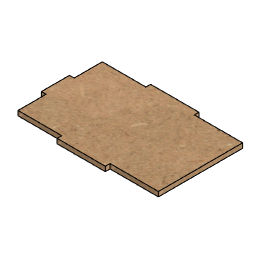
side step v13 (Autodesk Fusion 360 design; units mm, degrees)
Autodesk Fusion 360 part; units mm, degrees
sketch "Sketch1" plane through (0, 0, 0) normal (0, 0, 1) x (1, 0, 0)
  line L0 (-46.5, 30) -> (46.5, 30)
  line L1 (46.5, 30) -> (46.5, -30)
  line L2 (46.5, -30) -> (-46.5, -30)
  line L3 (-46.5, -30) -> (-46.5, 30)
  line L4 (-46.5, 30) -> (46.5, -30) construction
  line L5 (46.5, 30) -> (-46.5, -30) construction
  line L6 (-46.5, 30) -> (-15.5, 30)
  line L7 (-15.5, 30) -> (-15.5, 27)
  line L8 (-15.5, 27) -> (-46.5, 27)
  line L9 (-46.5, 27) -> (-46.5, 30)
  line L10 (-46.5, -30) -> (-15.5, -30)
  line L11 (-15.5, -30) -> (-15.5, -27)
  line L12 (-15.5, -27) -> (-46.5, -27)
  line L13 (-46.5, -27) -> (-46.5, -30)
  line L14 (46.5, 30) -> (15.5, 30)
  line L15 (15.5, 30) -> (15.5, 27)
  line L16 (15.5, 27) -> (46.5, 27)
  line L17 (46.5, 27) -> (46.5, 30)
  line L18 (46.5, -30) -> (15.5, -30)
  line L19 (15.5, -30) -> (15.5, -27)
  line L20 (15.5, -27) -> (46.5, -27)
  line L21 (46.5, -27) -> (46.5, -30)
  line L22 (46.5, 30) -> (43.5, 30)
  line L23 (43.5, 30) -> (43.5, 27)
  line L24 (43.5, 27) -> (46.5, 27)
  line L25 (46.5, 27) -> (46.5, 30)
  line L26 (46.5, -30) -> (43.5, -30)
  line L27 (43.5, -30) -> (43.5, -27)
  line L28 (43.5, -27) -> (46.5, -27)
  line L29 (46.5, -27) -> (46.5, -30)
  line L30 (-46.5, 27) -> (-43.5, 27)
  line L31 (-43.5, 27) -> (-43.5, 9)
  line L32 (-43.5, 9) -> (-46.5, 9)
  line L33 (-46.5, 9) -> (-46.5, 27)
  line L34 (-46.5, -27) -> (-43.5, -27)
  line L35 (-43.5, -27) -> (-43.5, -9)
  line L36 (-43.5, -9) -> (-46.5, -9)
  line L37 (-46.5, -9) -> (-46.5, -27)
  dimension "d1" = 93
  dimension "d2" = 60
  dimension "d3" = 31
  dimension "d4" = 3
  dimension "d5" = 31
  dimension "d6" = 3
  dimension "d7" = 31
  dimension "d8" = 3
  dimension "d9" = 31
  dimension "d10" = 3
  dimension "d11" = 3
  dimension "d12" = 3
  dimension "d13" = 3
  dimension "d14" = 3
  dimension "d15" = 3
  dimension "d16" = 18
  dimension "d17" = 3
  dimension "d18" = 18
  constraint horizontal L0
  constraint perpendicular L0 L1
  constraint parallel L0 L2
  constraint parallel L1 L3
  constraint coincident L4 origin
  constraint coincident L5 origin
  constraint horizontal L6
  constraint vertical L7
  constraint horizontal L8
  constraint vertical L9
  constraint horizontal L10
  constraint vertical L11
  constraint horizontal L12
  constraint vertical L13
  constraint horizontal L14
  constraint vertical L15
  constraint horizontal L16
  constraint vertical L17
  constraint horizontal L18
  constraint vertical L19
  constraint horizontal L20
  constraint vertical L21
  constraint horizontal L22
  constraint vertical L23
  constraint horizontal L24
  constraint vertical L25
  constraint horizontal L26
  constraint vertical L27
  constraint horizontal L28
  constraint vertical L29
  constraint horizontal L30
  constraint vertical L31
  constraint horizontal L32
  constraint vertical L33
  constraint horizontal L34
  constraint vertical L35
  constraint horizontal L36
  constraint vertical L37
  measures "d1" distance of L1.end L2.end
  measures "d2" distance of L0.end L1.end
  measures "d3" distance of L0.start L6.end
  measures "d4" distance of L0.start L8.end
  measures "d5" distance of L2.end L10.end
  measures "d6" distance of L2.end L12.end
  measures "d7" distance of L0.end L14.end
  measures "d8" distance of L0.end L16.end
  measures "d9" distance of L1.end L18.end
  measures "d10" distance of L1.end L20.end
  measures "d11" distance of L0.end L22.end
  measures "d12" distance of L0.end L16.end
  measures "d13" distance of L1.end L26.end
  measures "d14" distance of L1.end L20.end
  measures "d15" distance of L8.end L30.end
  measures "d16" distance of L8.end L32.end
  measures "d17" distance of L12.end L34.end
  measures "d18" distance of L12.end L36.end
extrude "Extrude1" add sketch "Sketch1" along normal blind 3 contours L0 L1 L2 L3 L7 L8 L11 L12 L15 L16 L19 L20 L24 L28 L31 L32 L35 L36
sketch "Sketch2" plane through (0, 0, 3) normal (0, 0, 1) x (-1, 0, 0)
  line L0 (-15.5, 30) -> (-15.5, 27)
  line L1 (-15.5, 27) -> (-46.5, 27)
  line L2 (-46.5, 27) -> (-46.5, -27)
  line L3 (-46.5, -27) -> (-15.5, -27)
  line L4 (-15.5, -27) -> (-15.5, -30)
  line L5 (-15.5, -30) -> (15.5, -30)
  line L6 (15.5, -30) -> (15.5, -27)
  line L7 (15.5, -27) -> (43.5, -27)
  line L8 (43.5, -27) -> (43.5, -9)
  line L9 (43.5, -9) -> (46.5, -9)
  line L10 (46.5, -9) -> (46.5, 9)
  line L11 (46.5, 9) -> (43.5, 9)
  line L12 (43.5, 9) -> (43.5, 27)
  line L13 (43.5, 27) -> (15.5, 27)
  line L14 (15.5, 27) -> (15.5, 30)
  line L15 (15.5, 30) -> (-15.5, 30)
